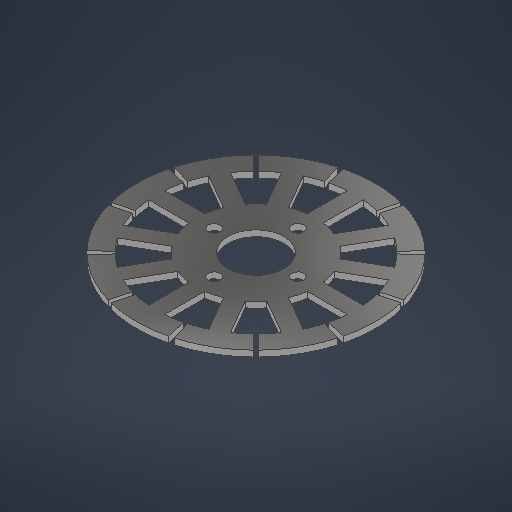
# Autodesk Inventor part: lamina_estator
Saved by Autodesk Inventor 2025 (Build 290162010, 162A)
## iProperties
Created: 2024-11-08
Part Number: lamina_estator
Material: Generic
Document SubType Name: Modeling
Designer: river
Density: 1 g/cm^3
Appearance: Default
Author: river
Autodesk Inventor part; units mm, degrees
ref_plane "YZ Plane" through (0, 0, 0) normal (1, 0, 0) x (0, 1, 0)
ref_plane "XZ Plane" through (0, 0, 0) normal (0, 1, 0) x (-1, 0, 0)
ref_plane "XY Plane" through (0, 0, 0) normal (0, 0, 1) x (1, 0, 0)
sketch "Sketch2" plane through (0, 0, 0) normal (0, 1, 0) x (-1, 0, 0)
  circle A0 centre (0, 0) radius 30
  circle A1 centre (0, 0) radius 50 construction
  circle A2 centre (0, 0) radius 60 construction
  line L0 (0, 0) -> (60, 0) construction
  line L1 (48.5148, 12.0961) -> (58.2177, 14.5153)
  line L2 (29.7321, 4) -> (49.8397, 4)
  line L3 (48.5148, -12.0961) -> (58.2177, -14.5153)
  line L4 (29.7321, -4) -> (49.8397, -4)
  arc A3 (58.2177, -14.5153) -> (58.2177, 14.5153) centre (0, 0) ccw
  arc A4 (49.8397, 4) -> (48.5148, 12.0961) centre (0, 0) ccw
  arc A5 (48.5148, -12.0961) -> (49.8397, -4) centre (0, 0) ccw
  point P0 (30, 0)
  dimension "d3" = 60
  dimension "d4" = 100
  dimension "d5" = 120
  dimension "d6" = 8
  dimension "d7" = 28
  constraints: 12 point on circle, 10 end point, 6 centre point, 4 symmetric about line, 3 coincident, 3 concentric, 2 horizontal, 2 line through centre
  measures "d3" diameter of A0
  measures "d4" diameter of A1
  measures "d5" diameter of A2
  measures "d6" distance between parallel lines of L4 L2
  measures "d7" angle of L3 L1
extrude "Extrusion1" add sketch "Sketch2" along normal blind 3 contours A0 L2 A4 L1 A3 L3 A5 L4
pattern_circular "Circular Pattern1" count 12 over 360 about axis through (0, -10, 0) along (0, 1, 0) of "Extrusion1"
extrude "Extrusion2" add sketch "Sketch2" along normal blind 3 contours A0
sketch "Sketch3" plane through (0, 3, 0) normal (0, 1, 0) x (1, 0, 0)
  circle A0 centre (-21, 0) radius 3
  line L0 (0, 0) -> (-21, 0) construction
  circle A1 centre (0, -21) radius 3
  circle A2 centre (21, 0) radius 3
  circle A3 centre (0, 0) radius 14
  circle A4 centre (0, 21) radius 3
  dimension "d15" = 21
  dimension "d16" = 6
  dimension "d19" = 360
  dimension "d21" = 28
  constraints: 5 centre point, 2 end point, 1 coincident, 1 horizontal, 9 other
  measures "d15" distance of L0.start L0.end
  measures "d16" diameter of A0
  measures "d21" diameter of A3
extrude "Extrusion3" cut sketch "Sketch3" against normal blind 3
body "Solid1"
